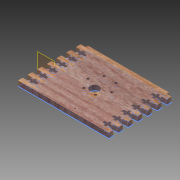
# Autodesk Inventor part: stepperMotorMountPlate01resized01
Saved by Autodesk Inventor 2013 (Build 170138000, 138)
## iProperties
Created: 2013-02-23
Part Number: stepperMotorMountPlate01resized01
Material: Wood (Birch)
Document SubType Name: Modeling
Designer: Nano
Density: 0.55 g/cm^3
Mass: 20.9125 g
Surface Area: 257.148 cm^2
Volume: 38.0226 cm^3
Author: Nano
Autodesk Inventor part; units mm, degrees
ref_plane "YZ Plane" through (0, 0, 0) normal (1, 0, 0) x (0, 1, 0)
ref_plane "XZ Plane" through (0, 0, 0) normal (0, 1, 0) x (-1, 0, 0)
ref_plane "XY Plane" through (0, 0, 0) normal (0, 0, 1) x (1, 0, 0)
sketch "Sketch1" plane through (0, 0, 0) normal (0, 1, 0) x (-1, 0, 0)
  line L0 (64.0604, 50.8) -> (-62.9396, 50.8)
  line L1 (-62.9396, 50.8) -> (-62.9396, -50.8)
  line L2 (-62.9396, -50.8) -> (64.0604, -50.8)
  line L3 (64.0604, -50.8) -> (64.0604, 50.8)
  line L4 (0, 0) -> (101.6, 0) construction
  line L5 (0, 50.8) -> (0, -50.8) construction
  line L6 (-58.3406, 0) -> (58.3406, 0) construction
  circle A0 centre (0, 0) radius 6
  circle A1 centre (-15.5097, -7.0044) radius 1.5875
  circle A2 centre (15.5097, -7.0044) radius 1.5875
  circle A3 centre (7.7597, 6.419) radius 1.5875
  circle A4 centre (7.7597, -20.4278) radius 1.5875
  circle A5 centre (-7.75, 6.4234) radius 1.5875
  circle A6 centre (-7.75, -20.4234) radius 1.5875
  arc A7 (1.7433, -2.4415) -> (-1.8557, -2.3572) centre (0, 0) ccw
  point P0 (0, 0)
  point P1 (0, 0)
  dimension "d1" = 127
  dimension "d2" = 101.6
  dimension "d31" = 12
  dimension "d32" = 0
  dimension "d33" = 3.175
  dimension "d34" = 17.018
  dimension "d35" = 3.175
  dimension "d36" = 17.018
  dimension "d37" = 3.175
  dimension "d38" = 3.175
  dimension "d39" = 10.0706
  dimension "d40" = 21.8519
  dimension "d41" = 15.5
  dimension "d42" = 15.5
  constraints: 14 end point, 8 centre point, 2 coincident, 2 horizontal, 2 parallel, 2 point on circle, 1 midpoint, 1 perpendicular, 1 vertical
  measures "d1" distance of L0.start L0.end
  measures "d2" distance of L1.end L0.end
  measures "d31" diameter of A0
  measures "d32" distance of point (0, 0) A0.centre
  measures "d33" diameter of A1
  measures "d34" distance of point (0, 0) A1.centre
  measures "d35" diameter of A2
  measures "d36" distance of point (0, 0) A2.centre
  measures "d37" diameter of A3
  measures "d38" diameter of A4
  measures "d39" distance of A3.centre point (0, 0)
  measures "d40" distance of A4.centre point (0, 0)
  measures "d41" distance of A4.centre A2.centre
  measures "d42" distance of A2.centre A3.centre
extrude "Extrusion1" add sketch "Sketch1" along normal blind 6.35
ref_plane "Work Plane1" through (-64.0604, 0, 0) normal (0, 0, 1) x (1, 0, 0)
sketch "Sketch4" plane through (0, 0, 0) normal (0, -1, 0) x (1, 0, 0)
  line L0 (-59.5312, 50.8) -> (59.5312, 50.8)
  line L1 (59.5312, 50.8) -> (59.5312, 41.0053)
  line L2 (59.5312, 41.0053) -> (-59.5312, 41.0053)
  line L3 (-59.5312, 41.0053) -> (-59.5312, 50.8)
  constraints: 8 end point, 2 parallel, 1 horizontal, 1 perpendicular
extrude "Extrusion4" cut sketch "Sketch4" against normal through all
sketch "Sketch5" plane through (0, 6.35, 0) normal (0, 1, 0) x (1, 0, 0)
  line L0 (-52.7198, 44.4492) -> (53.644, 44.4507)
  line L1 (-52.7198, 44.4492) -> (-52.7197, 41.2742)
  line L2 (-52.7197, 41.2742) -> (-59.0741, 41.2741)
  line L3 (-59.074, 34.9241) -> (-59.0741, 41.2741)
  line L4 (-59.074, 34.9241) -> (-52.7197, 34.9242)
  line L5 (-52.7197, 34.9242) -> (-52.7196, 33.3367)
  line L6 (-52.7196, 33.3367) -> (-49.9415, 33.3368)
  line L7 (-49.9415, 33.3368) -> (-49.9415, 35.718)
  line L8 (-49.9415, 35.718) -> (-46.7665, 35.7181)
  line L9 (-46.7665, 35.7181) -> (-46.7665, 33.3368)
  line L10 (-46.7665, 33.3368) -> (-42.687, 33.3369)
  line L11 (-42.687, 33.3369) -> (-42.687, 30.1619)
  line L12 (-42.687, 30.1619) -> (-46.7665, 30.1618)
  line L13 (-46.7665, 30.1618) -> (-46.7664, 27.7806)
  line L14 (-46.7664, 27.7806) -> (-49.9414, 27.7805)
  line L15 (-49.9414, 27.7805) -> (-49.9415, 30.1618)
  line L16 (-49.9415, 30.1618) -> (-52.7196, 30.1617)
  line L17 (-52.7196, 30.1617) -> (-52.7196, 28.5742)
  line L18 (-52.7196, 28.5742) -> (-59.0739, 28.5741)
  line L19 (-59.0738, 22.2241) -> (-59.0739, 28.5741)
  line L20 (-59.0738, 22.2241) -> (-52.7195, 22.2242)
  line L21 (-52.7195, 22.2242) -> (-52.7195, 20.6367)
  line L22 (-52.7195, 20.6367) -> (-49.9413, 20.6368)
  line L23 (-49.9413, 20.6368) -> (-49.9414, 23.018)
  line L24 (-49.9414, 23.018) -> (-46.7664, 23.0181)
  line L25 (-46.7664, 23.0181) -> (-46.7663, 20.6368)
  line L26 (-46.7663, 20.6368) -> (-42.6869, 20.6369)
  line L27 (-42.6869, 20.6369) -> (-42.6868, 17.4619)
  line L28 (-42.6868, 17.4619) -> (-46.7845, 17.4618)
  line L29 (-46.7845, 17.4618) -> (-46.7844, 15.0806)
  line L30 (-46.7844, 15.0806) -> (-49.9594, 15.0805)
  line L31 (-49.9594, 15.0805) -> (-49.9595, 17.4618)
  line L32 (-49.9595, 17.4618) -> (-52.7376, 17.4617)
  line L33 (-52.7376, 17.4617) -> (-52.7376, 15.8742)
  line L34 (-52.7376, 15.8742) -> (-59.0919, 15.8741)
  line L35 (-59.0918, 9.5241) -> (-59.0919, 15.8741)
  line L36 (-59.0918, 9.5241) -> (-52.7193, 9.5242)
  line L37 (-52.7193, 9.5242) -> (-52.7193, 7.9367)
  line L38 (-52.7193, 7.9367) -> (-49.9411, 7.9368)
  line L39 (-49.9411, 7.9368) -> (-49.9412, 10.318)
  line L40 (-49.9412, 10.318) -> (-46.7662, 10.3181)
  line L41 (-46.7662, 10.3181) -> (-46.7661, 7.9368)
  line L42 (-46.7661, 7.9368) -> (-42.6867, 7.9369)
  line L43 (-42.6867, 7.9369) -> (-42.6866, 4.7619)
  line L44 (-42.6866, 4.7619) -> (-46.7661, 4.7618)
  line L45 (-46.7661, 4.7618) -> (-46.7661, 2.3806)
  line L46 (-46.7661, 2.3806) -> (-49.9411, 2.3805)
  line L47 (-49.9411, 2.3805) -> (-49.9411, 4.7618)
  line L48 (-49.9411, 4.7618) -> (-52.7192, 4.7617)
  line L49 (-52.7192, 4.7617) -> (-52.7192, 3.1742)
  line L50 (-52.7192, 3.1742) -> (-59.0735, 3.1741)
  line L51 (-59.0734, -3.1759) -> (-59.0735, 3.1741)
  line L52 (-59.0734, -3.1759) -> (-52.7191, -3.1758)
  line L53 (-52.7191, -3.1758) -> (-52.7191, -4.7633)
  line L54 (-52.7191, -4.7633) -> (-49.941, -4.7632)
  line L55 (-49.941, -4.7632) -> (-49.941, -2.382)
  line L56 (-49.941, -2.382) -> (-46.766, -2.3819)
  line L57 (-46.766, -2.3819) -> (-46.766, -4.7632)
  line L58 (-46.766, -4.7632) -> (-42.6865, -4.7631)
  line L59 (-42.6865, -4.7631) -> (-42.6865, -7.9381)
  line L60 (-42.6865, -7.9381) -> (-46.7659, -7.9382)
  line L61 (-46.7659, -7.9382) -> (-46.7659, -10.3194)
  line L62 (-46.7659, -10.3194) -> (-49.9409, -10.3195)
  line L63 (-49.9409, -10.3195) -> (-49.9409, -7.9382)
  line L64 (-49.9409, -7.9382) -> (-52.719, -7.9383)
  line L65 (-52.719, -7.9383) -> (-52.719, -9.5258)
  line L66 (-52.719, -9.5258) -> (-59.0733, -9.5259)
  line L67 (-59.0732, -15.8759) -> (-59.0733, -9.5259)
  line L68 (-59.0732, -15.8759) -> (-52.7189, -15.8758)
  line L69 (-52.7189, -15.8758) -> (-52.7189, -17.4633)
  line L70 (-52.7189, -17.4633) -> (-49.9408, -17.4632)
  line L71 (-49.9408, -17.4632) -> (-49.9408, -15.082)
  line L72 (-49.9408, -15.082) -> (-46.7658, -15.0819)
  line L73 (-46.7658, -15.0819) -> (-46.7658, -17.4632)
  line L74 (-46.7658, -17.4632) -> (-42.6863, -17.4631)
  line L75 (-42.6863, -17.4631) -> (-42.6863, -20.6381)
  line L76 (-42.6863, -20.6381) -> (-46.7657, -20.6382)
  line L77 (-46.7657, -20.6382) -> (-46.7657, -23.0194)
  line L78 (-46.7657, -23.0194) -> (-49.9407, -23.0195)
  line L79 (-49.9407, -23.0195) -> (-49.9407, -20.6382)
  line L80 (-49.9407, -20.6382) -> (-52.7189, -20.6383)
  line L81 (-52.7189, -20.6383) -> (-52.7188, -22.2258)
  line L82 (-52.7188, -22.2258) -> (-59.0731, -22.2259)
  line L83 (-59.0731, -28.5759) -> (-59.0731, -22.2259)
  line L84 (-59.0731, -28.5759) -> (-52.7188, -28.5758)
  line L85 (-52.7188, -28.5758) -> (-52.7187, -30.1633)
  line L86 (-52.7187, -30.1633) -> (-49.9406, -30.1632)
  line L87 (-49.9406, -30.1632) -> (-49.9406, -27.782)
  line L88 (-49.9406, -27.782) -> (-46.7656, -27.7819)
  line L89 (-46.7656, -27.7819) -> (-46.7656, -30.1632)
  line L90 (-46.7656, -30.1632) -> (-42.6861, -30.1631)
  line L91 (-42.6861, -30.1631) -> (-42.6861, -33.3381)
  line L92 (-42.6861, -33.3381) -> (-46.7656, -33.3382)
  line L93 (-46.7656, -33.3382) -> (-46.7655, -35.7194)
  line L94 (-46.7655, -35.7194) -> (-49.9405, -35.7195)
  line L95 (-49.9405, -35.7195) -> (-49.9406, -33.3382)
  line L96 (-49.9406, -33.3382) -> (-52.7187, -33.3383)
  line L97 (-52.7187, -33.3383) -> (-52.7187, -34.9258)
  line L98 (-52.7187, -34.9258) -> (-59.073, -34.9259)
  line L99 (-59.0729, -41.2759) -> (-59.073, -34.9259)
  line L100 (-59.0729, -41.2759) -> (-52.7186, -41.2758)
  line L101 (-52.7186, -41.2758) -> (-52.7185, -44.4508)
  line L102 (53.6452, -44.4493) -> (-52.7185, -44.4508)
  line L103 (61.7256, -269.9687) -> (61.7256, 15.018) projected
  line L104 (61.7256, 15.018) -> (61.7256, 87.39) construction
  line L105 (0, 88.6989) -> (0, -326.401) construction
  line L106 (53.644, 44.4507) -> (53.644, 41.2757)
  line L107 (53.644, 41.2757) -> (59.9521, 41.2758)
  line L108 (59.9522, 34.9258) -> (59.9521, 41.2758)
  line L109 (59.9522, 34.9258) -> (53.6441, 34.9257)
  line L110 (53.6441, 34.9257) -> (53.6441, 33.3382)
  line L111 (53.6441, 33.3382) -> (50.866, 33.3382)
  line L112 (50.866, 33.3382) -> (50.866, 35.7195)
  line L113 (50.866, 35.7195) -> (47.691, 35.7194)
  line L114 (47.691, 35.7194) -> (47.691, 33.3382)
  line L115 (47.691, 33.3382) -> (43.6115, 33.3381)
  line L116 (43.6115, 33.3381) -> (43.6116, 30.1631)
  line L117 (43.6116, 30.1631) -> (47.691, 30.1632)
  line L118 (47.691, 30.1632) -> (47.6911, 27.7819)
  line L119 (47.6911, 27.7819) -> (50.8661, 27.782)
  line L120 (50.8661, 27.782) -> (50.866, 30.1632)
  line L121 (50.866, 30.1632) -> (53.6442, 30.1632)
  line L122 (53.6442, 30.1632) -> (53.6442, 28.5757)
  line L123 (53.6442, 28.5757) -> (59.9523, 28.5758)
  line L124 (59.9523, 22.2258) -> (59.9523, 28.5758)
  line L125 (59.9523, 22.2258) -> (53.6443, 22.2257)
  line L126 (53.6443, 22.2257) -> (53.6443, 20.6382)
  line L127 (53.6443, 20.6382) -> (50.8662, 20.6382)
  line L128 (50.8662, 20.6382) -> (50.8661, 23.0195)
  line L129 (50.8661, 23.0195) -> (47.6911, 23.0194)
  line L130 (47.6911, 23.0194) -> (47.6912, 20.6382)
  line L131 (47.6912, 20.6382) -> (43.6117, 20.6381)
  line L132 (43.6117, 20.6381) -> (43.6117, 17.4631)
  line L133 (43.6117, 17.4631) -> (47.7094, 17.4632)
  line L134 (47.7094, 17.4632) -> (47.7094, 15.0819)
  line L135 (47.7094, 15.0819) -> (50.8844, 15.082)
  line L136 (50.8844, 15.082) -> (50.8844, 17.4632)
  line L137 (50.8844, 17.4632) -> (53.6625, 17.4632)
  line L138 (53.6625, 17.4632) -> (53.6625, 15.8757)
  line L139 (53.6625, 15.8757) -> (59.9706, 15.8758)
  line L140 (59.9707, 9.5258) -> (59.9706, 15.8758)
  line L141 (59.9707, 9.5258) -> (53.6445, 9.5257)
  line L142 (53.6445, 9.5257) -> (53.6445, 7.9382)
  line L143 (53.6445, 7.9382) -> (50.8664, 7.9382)
  line L144 (50.8664, 7.9382) -> (50.8663, 10.3195)
  line L145 (50.8663, 10.3195) -> (47.6913, 10.3194)
  line L146 (47.6913, 10.3194) -> (47.6914, 7.9382)
  line L147 (47.6914, 7.9382) -> (43.6119, 7.9381)
  line L148 (43.6119, 7.9381) -> (43.6119, 4.7631)
  line L149 (43.6119, 4.7631) -> (47.6914, 4.7632)
  line L150 (47.6914, 4.7632) -> (47.6914, 2.3819)
  line L151 (47.6914, 2.3819) -> (50.8664, 2.382)
  line L152 (50.8664, 2.382) -> (50.8664, 4.7632)
  line L153 (50.8664, 4.7632) -> (53.6445, 4.7632)
  line L154 (53.6445, 4.7632) -> (53.6445, 3.1757)
  line L155 (53.6445, 3.1757) -> (59.9526, 3.1758)
  line L156 (59.9527, -3.1742) -> (59.9526, 3.1758)
  line L157 (59.9527, -3.1742) -> (53.6446, -3.1743)
  line L158 (53.6446, -3.1743) -> (53.6447, -4.7618)
  line L159 (53.6447, -4.7618) -> (50.8665, -4.7618)
  line L160 (50.8665, -4.7618) -> (50.8665, -2.3805)
  line L161 (50.8665, -2.3805) -> (47.6915, -2.3806)
  line L162 (47.6915, -2.3806) -> (47.6915, -4.7618)
  line L163 (47.6915, -4.7618) -> (43.6121, -4.7619)
  line L164 (43.6121, -4.7619) -> (43.6121, -7.9369)
  line L165 (43.6121, -7.9369) -> (47.6916, -7.9368)
  line L166 (47.6916, -7.9368) -> (47.6916, -10.3181)
  line L167 (47.6916, -10.3181) -> (50.8666, -10.318)
  line L168 (50.8666, -10.318) -> (50.8666, -7.9368)
  line L169 (50.8666, -7.9368) -> (53.6447, -7.9368)
  line L170 (53.6447, -7.9368) -> (53.6447, -9.5243)
  line L171 (53.6447, -9.5243) -> (59.9528, -9.5242)
  line L172 (59.9529, -15.8742) -> (59.9528, -9.5242)
  line L173 (59.9529, -15.8742) -> (53.6448, -15.8743)
  line L174 (53.6448, -15.8743) -> (53.6448, -17.4618)
  line L175 (53.6448, -17.4618) -> (50.8667, -17.4618)
  line L176 (50.8667, -17.4618) -> (50.8667, -15.0805)
  line L177 (50.8667, -15.0805) -> (47.6917, -15.0806)
  line L178 (47.6917, -15.0806) -> (47.6917, -17.4618)
  line L179 (47.6917, -17.4618) -> (43.6122, -17.4619)
  line L180 (43.6122, -17.4619) -> (43.6123, -20.6369)
  line L181 (43.6123, -20.6369) -> (47.6918, -20.6368)
  line L182 (47.6918, -20.6368) -> (47.6918, -23.0181)
  line L183 (47.6918, -23.0181) -> (50.8668, -23.018)
  line L184 (50.8668, -23.018) -> (50.8668, -20.6368)
  line L185 (50.8668, -20.6368) -> (53.6449, -20.6368)
  line L186 (53.6449, -20.6368) -> (53.6449, -22.2243)
  line L187 (53.6449, -22.2243) -> (59.953, -22.2242)
  line L188 (59.9531, -28.5742) -> (59.953, -22.2242)
  line L189 (59.9531, -28.5742) -> (53.645, -28.5743)
  line L190 (53.645, -28.5743) -> (53.645, -30.1618)
  line L191 (53.645, -30.1618) -> (50.8669, -30.1618)
  line L192 (50.8669, -30.1618) -> (50.8669, -27.7805)
  line L193 (50.8669, -27.7805) -> (47.6919, -27.7806)
  line L194 (47.6919, -27.7806) -> (47.6919, -30.1618)
  line L195 (47.6919, -30.1618) -> (43.6124, -30.1619)
  line L196 (43.6124, -30.1619) -> (43.6125, -33.3369)
  line L197 (43.6125, -33.3369) -> (47.6919, -33.3368)
  line L198 (47.6919, -33.3368) -> (47.692, -35.7181)
  line L199 (47.692, -35.7181) -> (50.867, -35.718)
  line L200 (50.867, -35.718) -> (50.8669, -33.3368)
  line L201 (50.8669, -33.3368) -> (53.6451, -33.3368)
  line L202 (53.6451, -33.3368) -> (53.6451, -34.9243)
  line L203 (53.6451, -34.9243) -> (59.9532, -34.9242)
  line L204 (59.9533, -41.2742) -> (59.9532, -34.9242)
  line L205 (59.9533, -41.2742) -> (53.6452, -41.2743)
  line L206 (53.6452, -41.2743) -> (53.6452, -44.4493)
  line L207 (-59.5312, -41.0053) -> (59.5312, -41.0053) projected
  ellipse E0 centre (-53.2862, 17.4229) end of major axis (-53.3662, -52.4271) minor radius 0.546 (-52.7431, 15.1202) -> (-53.8349, 14.6815) ccw projected
  ellipse E1 centre (-59.636, 17.4301) end of major axis (-59.556, 87.2801) minor radius 0.546 (-59.0929, 15.1275) -> (-60.1847, 14.6887) ccw projected
  point P0 (-58.3406, -41.0053)
  point P1 (58.3406, -41.0053)
  constraints: 410 end point, 1 vertical, 6 other
extrude "Extrusion7" cut sketch "Sketch5" against normal blind 25.4 contours L0 L106 L107 L108 L109 L110 L111 L112 L113 L114 L115 L116 L117 L118 L119 L120 L121 L122 L123 L124 L125 L126 L127 L128 L129 L130 L131 L132 L133 L134 L135 L136 L137 L138 L139 L140 L141 L142 L143 L144 L145 L146 L147 L148 L149 L150 L151 L152 L153 L154 L155 L156 L157 L158 L159 L160 L161 L162 L163 L164 L165 L166 L167 L168 L169 L170 L171 L172 L173 L174 L175 L176 L177 L178 L179 L180 L181 L182 L183 L184 L185 L186 L187 L188 L189 L190 L191 L192 L193 L194 L195 L196 L197 L198 L199 L200 L201 L202 L203 L204 L205 L206 L102 L101 L100 L99 L98 L97 L96 L95 L94 L93 L92 L91 L90 L89 L88 L87 L86 L85 L84 L83 L82 L81 L80 L79 L78 L77 L76 L75 L74 L73 L72 L71 L70 L69 L68 L67 L66 L65 L64 L63 L62 L61 L60 L59 L58 L57 L56 L55 L54 L53 L52 L51 L50 L49 L48 L47 L46 L45 L44 L43 L42 L41 L40 L39 L38 L37 L36 L35 L34 L33 L32 L31 L30 L29 L28 L27 L26 L25 L24 L23 L22 L21 L20 E0 L18 L17 L16 L15 L14 L13 L12 L11 L10 L9 L8 L7 L6 L5 L4 L2 L1 | E0 L4 L2 | E0 L4 L3 L2 | E0 L20 L18 | E0 L20 L19 L18 keep common part
equation "\"d42\" = d41"
body "Solid1"
